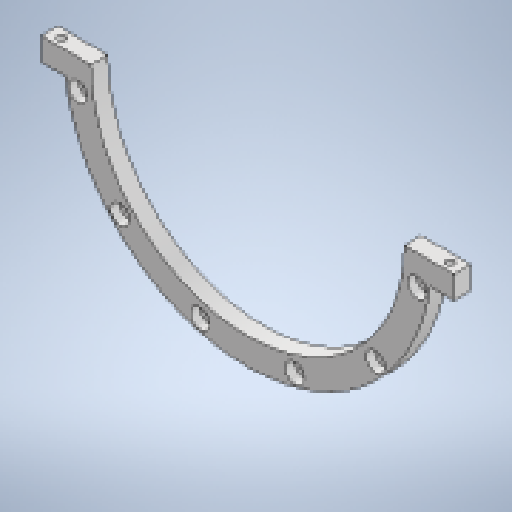
# Autodesk Inventor part: ДМФ 093 Постель КОРМА v2.0_CPY
Saved by Autodesk Inventor 2026.2 (Build 302298010, 298A)
## iProperties
Created: 2024-04-28
Part Number: ДМФ 093 Постель КОРМА v2.0_CPY
Material: Nylon 6
Document SubType Name: Sheet Metal
Designer: admin
Stock Number: Постель_Корма
Density: 1.12 g/cm^3
Sheet Metal Rule: Default
Sheet Metal Width: 0,000 mm
Sheet Metal Length: 0,000 mm
Sheet Metal Area: 0,000 mm^2
Appearance: Default
Author: pokla
Autodesk Inventor part; units mm, degrees
ref_plane "YZ Plane" through (0, 0, 0) normal (1, 0, 0) x (0, 1, 0)
ref_plane "XZ Plane" through (0, 0, 0) normal (0, 1, 0) x (-1, 0, 0)
ref_plane "XY Plane" through (0, 0, 0) normal (0, 0, 1) x (1, 0, 0)
sketch "Sketch1" plane through (0, 0, 0) normal (0, 0, 1) x (1, 0, 0)
  circle A0 centre (0, 0) radius 220 construction
  circle A1 centre (0, 0) radius 205
  circle A2 centre (0, 0) radius 240
  line L0 (-205, 0) -> (-205, 80) construction
  line L1 (-205, 80) -> (-240, 80) construction
  line L2 (-240, 80) -> (-240, 0) construction
  line L3 (-205, 0) -> (-240, 0)
  line L4 (-240, 0) -> (-270, 0)
  line L5 (-270, 0) -> (-270, -30)
  line L6 (-270, -30) -> (-238.1176, -30)
  line L7 (-1.5, -238) -> (1.5, -238)
  line L8 (1.5, -238) -> (1.5, -280)
  line L9 (1.5, -280) -> (-1.5, -280)
  line L10 (-1.5, -280) -> (-1.5, -238)
  line L11 (0, -238) -> (0, -205)
  line L12 (-1.5, -280) -> (-30, -280)
  line L13 (-30, -280) -> (-30, -238.1176)
  line L14 (0, -238) -> (0, -240)
  point P0 (0, -280)
  point P1 (-1.5, -239.9953)
  point P2 (1.5, -239.9953)
  dimension "d26" = 80
  dimension "d40" = 30
  dimension "d41" = 30
  dimension "d74" = 410
  dimension "d75" = 3
  dimension "d76" = 42
  dimension "d77" = 30
  dimension "d78" = 2
  dimension "d98" = 480
  dimension "d99" = 440
  constraints: 30 end point, 6 perpendicular, 6 point on circle, 3 centre point, 3 coincident, 3 horizontal, 3 vertical, 2 midpoint, 2 parallel, 2 tangent, 1 point on line, 1 vertical alignment
  measures "d26" distance of L0.start L0.end
  measures "d40" distance of L2.end L4.end
  measures "d41" distance of L4.end L5.end
  measures "d74" diameter of A1
  measures "d75" distance of L7.start L7.end
  measures "d76" distance of L9.end L7.start
  measures "d77" distance from line of point (0, -280) L13
  measures "d78" distance of L11.start L14.end
  measures "d98" diameter of A2
  measures "d99" diameter of A0
extrude "Extrusion1" add sketch "Sketch1" against normal blind 22 contours A1 L11 L7 L10 A2 L3 | A2 L6 L5 L4 | L14 A2 L10 L7
sketch "Sketch10" plane through (-270, -30, 0) normal (0, -1, 0) x (1, 0, 0)
  line L0 (0, 0) -> (31.8824, 0) projected
  line L1 (0, 0) -> (0, -22) projected
  line L2 (31.8824, -22) -> (0, -22) projected
  line L3 (31.8824, 0) -> (31.8824, -22) projected
  circle A0 centre (15.9412, -11) radius 5.5
  line L4 (0, 0) -> (0, -22) projected
  line L5 (0, 0) -> (31.8824, 0) projected
  point P0 (270, 0)
  point P1 (0, -11)
  point P2 (15.9412, 0)
  dimension "d79" = 11
  constraints: 2 midpoint, 1 centre point, 1 horizontal alignment, 1 vertical alignment
  measures "d79" diameter of A0
extrude "Extrusion9" cut sketch "Sketch10" against normal through all contours A0
mirror "Mirror3" about plane through (0, 0, 0) normal (1, 0, 0) of "Extrusion1", "Extrusion9"
sketch "Sketch12" plane through (0, 0, 0) normal (0, 0, 1) x (1, 0, 0)
  line L0 (0, 0) -> (-225, 0) construction
  line L1 (0, 0) -> (-221.5817, -39.0708) construction
  circle A0 centre (0, 0) radius 225 construction
  dimension "d86" = 10
  dimension "d87" = 450
  constraints: 4 end point, 2 coincident, 2 point on circle, 1 centre point, 1 horizontal
  measures "d86" angle of L1 L0
  measures "d87" diameter of A0
hole "Hole4" at (-221.5817, -39.0708, 0) direction (0, 0, -1) diameter 11 end through all counterbore diameter 26 counterbore depth 12
pattern_circular "Circular Pattern5" count 6 over 160 about axis through (0, 0, -10) along (0, 0, 1) of "Hole4"
equation "\"d41\" = d40"
equation "\"d77\" = d41"
equation "\"d93\" = Thickness"
equation "\"BendReliefDepth\" = 0.5 * Thickness"
equation "\"Thickness\" = 30"
body "Solid1"
